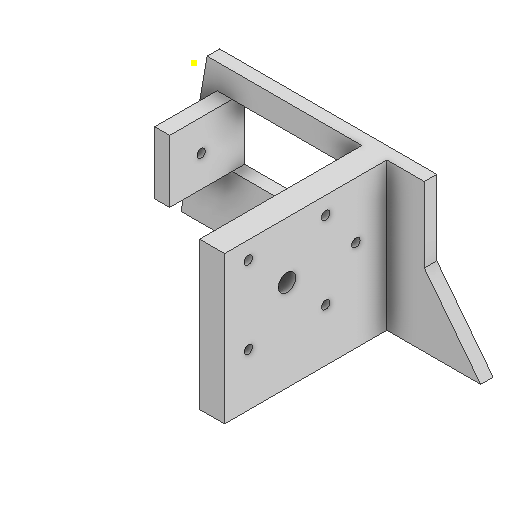
# Autodesk Inventor part: podstawka pod silnik
Saved by Autodesk Inventor 2025.1 (Build 291241000, 241)
## iProperties
Created: 2025-03-27
Part Number: podstawka pod silnik
Material: Ogólny
Document SubType Name: Modeling
Designer: Maciej
Density: 1 g/cm^3
Appearance: Domyślna
Author: Maciej
Autodesk Inventor part; units mm, degrees
ref_plane "YZ Plane" through (0, 0, 0) normal (1, 0, 0) x (0, 1, 0)
ref_plane "XZ Plane" through (0, 0, 0) normal (0, 1, 0) x (-1, 0, 0)
ref_plane "XY Plane" through (0, 0, 0) normal (0, 0, 1) x (1, 0, 0)
sketch "Szkic1" plane through (0, 0, 0) normal (0, 0, 1) x (1, 0, 0)
  line L0 (0, 0) -> (120, 0)
  line L1 (0, 0) -> (10.4189, 59.0885)
  line L2 (0, 0) -> (60, 0) construction
  line L3 (120, 0) -> (97.4189, 29.0885)
  line L4 (10.4189, 59.0885) -> (70.4189, 59.0885)
  line L5 (10.4189, 59.0885) -> (70.4189, 59.0885) construction
  line L6 (97.4189, 29.0885) -> (97.4189, 59.0885)
  line L7 (97.4189, 59.0885) -> (70.4189, 59.0885)
  line L8 (20.4189, 49.0885) -> (70.4189, 49.0885)
  line L9 (70.4189, 49.0885) -> (70.4189, 24.0885)
  line L10 (70.4189, 24.0885) -> (20.4189, 24.0885)
  line L11 (20.4189, 24.0885) -> (20.4189, 49.0885)
  line L12 (20.4189, 49.0885) -> (14.4189, 49.0885)
  line L13 (14.4189, 49.0885) -> (14.4189, 24.0885)
  line L14 (14.4189, 24.0885) -> (20.4189, 24.0885)
  line L15 (20.4189, 24.0885) -> (20.4189, 49.0885)
  line L16 (70.4189, 49.0885) -> (80.4189, 49.0885)
  line L17 (80.4189, 49.0885) -> (80.4189, 24.0885)
  line L18 (80.4189, 24.0885) -> (70.4189, 24.0885)
  line L19 (70.4189, 24.0885) -> (70.4189, 49.0885)
  dimension "d0" = 120
  dimension "d1" = 60
  dimension "d2" = 80
  dimension "d4" = 60
  dimension "d5" = 0
  dimension "d6" = 50
  dimension "d7" = 25
  dimension "d8" = 10
  dimension "d9" = 10
  dimension "d10" = 6
  dimension "d11" = 10
  dimension "d23" = 27
  dimension "d24" = 30
  constraints: 40 end point, 7 horizontal, 6 parallel, 5 perpendicular, 2 equal length, 2 point on line
  measures "d0" distance of L0.start L0.end
  measures "d1" distance of L0.start L1.end
  measures "d2" angle of L2 L1
  measures "d4" distance of L1.end L4.end
  measures "d5" distance between parallel lines of L4 L5
  measures "d6" distance of L9.end L10.end
  measures "d7" distance of L8.end L9.end
  measures "d8" distance from line of L4 L8.start
  measures "d9" horizontal distance of L1.end L8.start
  measures "d10" distance of L14.end L13.end
  measures "d11" distance of L17.end L18.end
  measures "d23" distance of L6.end L5.end
  measures "d24" distance of L3.end L6.end
extrude "Wyciągnięcie proste1" add sketch "Szkic1" along normal blind 5
extrude "Wyciągnięcie proste2" add sketch "Szkic1" along normal blind 30 contours L11 L14 L13 L12
extrude "Wyciągnięcie proste3" add sketch "Szkic1" along normal blind 50 contours L16 L17 L18 L9
sketch "Szkic2" plane through (70.4189, 49.0885, 5) normal (0, 1, 0) x (1, 0, 0)
  point P0 (-70.4189, 5)
sketch "Szkic3" plane through (70.4189, 49.0885, 5) normal (0, 1, 0) x (1, 0, 0)
  line L0 (0, 0) -> (0, -45) projected
  line L1 (-70.4189, 0) -> (49.5811, 0) projected
  line L2 (0, -45) -> (10, -45)
  line L3 (10, -45) -> (10, 0)
  line L4 (10, 0) -> (0, 0)
  line L5 (0, 0) -> (0, -45)
  point P0 (-70.4189, 5)
  dimension "d18" = 10
  constraints: 8 end point, 2 parallel, 1 horizontal, 1 perpendicular, 1 point on line
  measures "d18" distance of L4.end L3.end
extrude "Wyciągnięcie proste4" add sketch "Szkic3" along normal blind 10
sketch "Szkic4" plane through (70.4189, 24.0885, 5) normal (0, -1, 0) x (1, 0, 0)
  line L0 (0, 45) -> (10, 45) projected
  line L1 (0, 0) -> (0, -5) projected
  line L2 (10, 45) -> (0, 45)
  line L3 (0, 45) -> (0, 0)
  line L4 (0, 0) -> (10, 0)
  line L5 (10, 0) -> (10, 45)
  point P0 (-70.4189, -5)
  constraints: 8 end point, 2 parallel, 1 horizontal, 1 perpendicular
extrude "Wyciągnięcie proste5" add sketch "Szkic4" along normal up to surface (24.0885 mm away)
sketch "Szkic5" plane through (0, 0, 50) normal (0, 0, 1) x (1, 0, 0)
  line L0 (70.4189, 49.0885) -> (70.4189, 59.0885) projected
  line L1 (80.4189, 59.0885) -> (80.4189, 0) projected
  line L2 (70.4189, 59.0885) -> (80.4189, 59.0885)
  line L3 (80.4189, 59.0885) -> (80.4189, 0)
  line L4 (80.4189, 0) -> (70.4189, 0)
  line L5 (70.4189, 0) -> (70.4189, 59.0885)
  point P0 (0, 0)
  constraints: 8 end point, 2 parallel, 1 horizontal, 1 perpendicular
extrude "Wyciągnięcie proste6" add sketch "Szkic5" along normal blind 20
sketch "Szkic6" plane through (70.4189, 24.0885, 0) normal (-1, 0, 0) x (0, 0, 1)
  line L0 (5, 35) -> (70, 35) projected
  line L1 (30, 25) -> (30, 0) projected
  point P0 (0, -24.0885)
  point P1 (45, 12.5)
  point P2 (30, 12.5)
  dimension "d27" = 22.5
  dimension "d28" = 15
  constraints: 1 midpoint
  measures "d27" distance from line of L0 point (45, 12.5)
  measures "d28" distance of point (30, 12.5) point (45, 12.5)
hole "Otwór1" at (70.4189, 36.5885, 45) direction (1, 0, 0) diameter 7 end through all
sketch "Szkic7" plane through (80.4189, 0, 5) normal (1, 0, 0) x (0, 0, -1)
  line L0 (0, 59.0885) -> (-65, 59.0885) projected
  line L1 (0, 0) -> (0, 24.0885) projected
  line L2 (-65, 59.0885) -> (0, 59.0885)
  line L3 (0, 59.0885) -> (0, 0)
  line L4 (0, 0) -> (-65, 0)
  line L5 (-65, 0) -> (-65, 59.0885)
  circle A0 centre (-40, 36.5885) radius 3.5 projected
  circle A1 centre (-40, 36.5885) radius 3.5
  point P0 (5, 0)
  constraints: 8 end point, 2 parallel, 1 centre point, 1 coincident, 1 horizontal, 1 perpendicular
extrude "Wyciągnięcie proste7" add sketch "Szkic7" along normal blind 2
sketch "Szkic8" plane through (70.4189, 24.0885, 0) normal (-1, 0, 0) x (0, 0, 1)
  line L0 (5, 35) -> (70, 35) projected
  line L1 (5, -24.0885) -> (70, -24.0885) projected
  line L2 (5, 35) -> (70, 35)
  line L3 (70, 35) -> (70, -24.0885)
  line L4 (70, -24.0885) -> (5, -24.0885)
  line L5 (5, -24.0885) -> (5, 35)
  line L6 (5, 35) -> (70, 35)
  line L7 (70, 35) -> (70, -24.0885)
  line L8 (70, -24.0885) -> (5, -24.0885)
  line L9 (5, -24.0885) -> (5, 35)
  circle A0 centre (45, 12.5) radius 3.5 projected
  circle A1 centre (45, 12.5) radius 3.5
  point P0 (0, -24.0885)
  point P1 (70, 35)
  constraints: 16 end point, 4 parallel, 2 horizontal, 2 perpendicular, 1 centre point, 1 coincident
extrude "Wyciągnięcie proste8" cut sketch "Szkic8" against normal blind 2
sketch "Szkic9" plane through (82.4189, 0, 5) normal (1, 0, 0) x (0, 0, -1)
  circle A0 centre (-40, 36.5885) radius 3.5 projected
  point P0 (5, 0)
  point P1 (-55.5, 52.0885)
  point P2 (-24.5, 52.0885)
  point P3 (-24.5, 52.0885)
  point P4 (-24.5, 21.0885)
  point P5 (-55.5, 21.0885)
  dimension "d40" = 31
  dimension "d41" = 31
  dimension "d42" = 31
  dimension "d43" = 31
  dimension "d44" = 15.5
  dimension "d45" = 15.5
  constraints: 1 coincident
  measures "d40" distance of point (-24.5, 52.088) point (-55.5, 52.088)
  measures "d41" distance of point (-24.5, 52.088) point (-24.5, 21.088)
  measures "d42" distance of point (-55.5, 21.088) point (-55.5, 52.088)
  measures "d43" distance of point (-55.5, 21.088) point (-24.5, 21.088)
  measures "d44" horizontal distance of A0.centre point (-24.5, 52.088)
  measures "d45" horizontal distance of A0.centre point (-24.5, 52.088)
hole "Otwór2" at (82.4189, 52.0885, 60.5) at (82.4189, 52.0885, 29.5) at (82.4189, 21.0885, 60.5) at (82.4189, 21.0885, 29.5) direction (-1, 0, 0) diameter 3.4 end through all clearance for "Śruba ze łbem stożkowym ISO 2009/7046" size "M3" standard "ISO"
sketch "Szkic10" plane through (14.4189, 24.0885, 5) normal (-1, 0, 0) x (0, 0, 1)
  point P0 (-5, -24.0885)
  point P1 (12.3965, 12.5)
hole "Otwór3" at (14.4189, 36.5885, 17.3965) direction (1, 0, 0) diameter 3.4 end through all clearance for "Śruba ze łbem stożkowym ISO 2009/7046" size "M3" standard "ISO"
equation "\"d41\" = d40"
equation "\"d42\" = d40"
equation "\"d43\" = d40"
